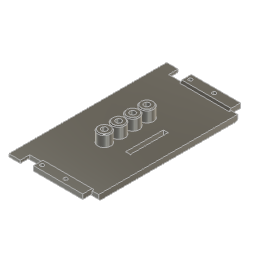
Case_Passthrough_v4 (Autodesk Fusion 360 design; units mm, degrees)
Autodesk Fusion 360 part; units mm, degrees
note: some values were not read from the file. Set by a fixed rule: which sketch regions a step uses.
sketch "Sketch1" plane through (0, 0, 0) normal (0, 0, 1) x (1, 0, 0)
  line L0 (0, 0) -> (-85, 0)
  line L1 (-85, 0) -> (-85, 147)
  line L2 (-85, 147) -> (0, 147)
  line L3 (0, 147) -> (0, 0)
  line L4 (-85, 0) -> (-85, 73.5)
  line L5 (-85, 73.5) -> (-85, 152)
  line L6 (-85, 73.5) -> (-85, -5)
  line L7 (-85, 152) -> (0, 152)
  line L8 (-85, -5) -> (0, -5)
  line L9 (-85, 152) -> (-55, 152)
  line L10 (-85, 152) -> (-30, 152)
  circle A0 centre (-55, 152) radius 2
  circle A1 centre (-30, 152) radius 2
  line L11 (-55, 152) -> (-55, -5)
  line L12 (-30, 152) -> (-30, -5)
  circle A2 centre (-55, -5) radius 2
  circle A3 centre (-30, -5) radius 2
  line L13 (-85, 147) -> (-73, 147)
  line L14 (-85, 147) -> (-59, 147)
  line L15 (-85, 147) -> (-7, 147)
  line L16 (-85, 147) -> (0, 147)
  line L17 (0, 147) -> (0, 157)
  line L18 (0, 157) -> (-85, 157)
  line L19 (-85, 157) -> (-85, 147)
  line L20 (-85, 0) -> (0, 0)
  line L21 (0, 0) -> (0, -10)
  line L22 (0, -10) -> (-85, -10)
  line L23 (-85, -10) -> (-85, 0)
  line L24 (-73, 147) -> (-73, -10)
  line L25 (-73, 147) -> (-73, 157)
  line L26 (-59, 147) -> (-59, 157)
  line L27 (-59, 147) -> (-59, -10)
  line L28 (-7, 147) -> (-7, 157)
  line L29 (-7, 147) -> (-7, -10)
  dimension "d1" = 85
  dimension "d2" = 147
  dimension "d3" = 78.5
  dimension "d4" = 78.5
  dimension "d5" = 30
  dimension "d6" = 55
  dimension "d7" = 4
  dimension "d8" = 4
  dimension "d9" = 4
  dimension "d10" = 4
  dimension "d11" = 12
  dimension "d12" = 26
  dimension "d13" = 78
  constraint horizontal L0
  constraint vertical L1
  constraint horizontal L2
  constraint vertical L3
  constraint coincident L0.start L3.end
  constraint midpoint L1 L4.end
  constraint perpendicular L2 L5
  constraint parallel L4 L6
  constraint perpendicular L5 L7
  constraint perpendicular L6 L8
  constraint perpendicular L5 L9
  constraint perpendicular L5 L10
  constraint coincident L9.end A0.centre
  constraint coincident L10.end A1.centre
  constraint coincident L8 L11.end
  constraint perpendicular L8 L11
  constraint coincident L8 L12.end
  constraint perpendicular L8 L12
  constraint coincident L11.end A2.centre
  constraint coincident L12.end A3.centre
  constraint perpendicular L1 L13
  constraint perpendicular L11 L14
  constraint perpendicular L12 L15
  constraint horizontal L16
  constraint vertical L17
  constraint horizontal L18
  constraint vertical L19
  constraint horizontal L20
  constraint vertical L21
  constraint horizontal L22
  constraint vertical L23
  constraint coincident L22 L24.end
  constraint perpendicular L22 L24
  constraint coincident L18 L25.end
  constraint perpendicular L18 L25
  constraint coincident L18 L26.end
  constraint perpendicular L18 L26
  constraint coincident L22 L27.end
  constraint perpendicular L22 L27
  constraint coincident L18 L28.end
  constraint perpendicular L18 L28
  constraint coincident L22 L29.end
  constraint perpendicular L22 L29
  measures "d1" distance of L0.start L0.end
  measures "d2" distance of L0.start L2.end
  measures "d3" distance of L4.end L5.end
  measures "d4" distance of L4.end L6.end
  measures "d5" distance of L5.end L9.end
  measures "d6" distance of L5.end L10.end
  measures "d7" diameter of A0
  measures "d8" diameter of A1
  measures "d9" diameter of A2
  measures "d10" diameter of A3
  measures "d11" distance of L1.end L13.end
  measures "d12" distance of L1.end L14.end
  measures "d13" distance of L1.end L15.end
extrude "Extrude1" add sketch "Sketch1" along normal blind 3 contours L0 L2 L3 L16 L20 L29 | L0 L8 L12 A3 L20 L29 | L0 L2 L12 L15 L16 L20 L29 | L0 L8 L11 L12 A2 A3 L20 | L0 L2 L11 L12 L15 L16 L20 | L2 L7 A1 L12 L15 L16 L28 | L8 A2 A3 L22 L27 L29 | L0 L8 L11 A2 L20 L27 | L0 L2 L11 L15 L16 L20 L27 | L2 L7 L10 A0 A1 L11 L12 L15 L16 | L7 L9 L10 A0 A1 L18 L26 L28 | L0 L2 L14 L15 L16 L20 L24 L27 | L2 L7 L9 L10 A0 L11 L15 L16 L26 | L0 L6 L8 L20 L23 L24 | L0 L1 L2 L4 L5 L6 L13 L14 L15 L16 L20 L24 | L8 L22 L23 L24 | L2 L5 L7 L9 L10 L13 L14 L15 L16 L19 L25 | L7 L9 L10 L18 L19 L25
sketch "Sketch2" plane through (0, 0, 0) normal (0, 0, 1) x (1, 0, 0)
extrude "Extrude2" add sketch "Sketch1" against normal blind 3 contours L0 L2 L3 L16 L20 L29 | L0 L2 L12 L15 L16 L20 L29 | L0 L2 L11 L12 L15 L16 L20 | L0 L2 L11 L15 L16 L20 L27 | L0 L2 L14 L15 L16 L20 L24 L27 | L0 L1 L2 L4 L5 L6 L13 L14 L15 L16 L20 L24
sketch "Sketch3" plane through (0, 0, 0) normal (0, 0, 1) x (1, 0, 0)
sketch "Sketch4" plane through (0, 0, -3) normal (0, 0, -1) x (1, 0, 0)
  line L0 (-85, 0) -> (-85, -147)
  line L1 (-85, -147) -> (0, -147)
  line L2 (0, -147) -> (0, 0)
  line L3 (0, 0) -> (-85, 0)
  line L4 (-85, 0) -> (-75, 0)
  line L5 (-75, 0) -> (-75, -10)
  line L6 (-75, -10) -> (-85, -10)
  line L7 (-85, -10) -> (-85, 0)
  line L8 (0, -147) -> (-10, -147)
  line L9 (-10, -147) -> (-10, -137)
  line L10 (-10, -137) -> (0, -137)
  line L11 (0, -137) -> (0, -147)
  line L12 (-75, -10) -> (-10, -10)
  line L13 (-10, -10) -> (-10, -137)
  line L14 (-10, -137) -> (-75, -137)
  line L15 (-75, -137) -> (-75, -10)
  dimension "d18" = 10
  dimension "d19" = 10
  dimension "d20" = 10
  dimension "d21" = 10
  constraint horizontal L4
  constraint vertical L5
  constraint horizontal L6
  constraint vertical L7
  constraint coincident L0.start L3.end
  constraint horizontal L8
  constraint vertical L9
  constraint horizontal L10
  constraint vertical L11
  constraint coincident L1.end L2.start
  constraint horizontal L12
  constraint vertical L13
  constraint horizontal L14
  constraint vertical L15
  measures "d18" distance of L0.start L4.end
  measures "d19" distance of L0.start L6.end
  measures "d20" distance of L1.end L8.end
  measures "d21" distance of L1.end L10.end
extrude "Extrude3" cut sketch "Sketch4" against normal blind 3 contours L12 L13 L14 L15
sketch "Sketch5" plane through (0, 0, 3) normal (0, 0, 1) x (-1, 0, 0)
  circle A0 centre (55, 5) radius 2
  circle A1 centre (55, -152) radius 2
  circle A2 centre (30, -152) radius 2
  circle A3 centre (30, 5) radius 2
  line L0 (73, 0) -> (59, 0)
  line L1 (59, 0) -> (59, 10)
  line L2 (59, 10) -> (7, 10)
  line L3 (7, 10) -> (7, 0)
  line L4 (7, 0) -> (0, 0)
  line L5 (0, 0) -> (0, -147)
  line L6 (0, -147) -> (7, -147)
  line L7 (7, -147) -> (7, -157)
  line L8 (7, -157) -> (59, -157)
  line L9 (59, -157) -> (59, -147)
  line L10 (59, -147) -> (73, -147)
  line L11 (73, -147) -> (73, -157)
  line L12 (73, -157) -> (85, -157)
  line L13 (85, -157) -> (85, 10)
  line L14 (85, 10) -> (73, 10)
  line L15 (73, 10) -> (73, 0)
  line L16 (0, -25) -> (45, -25)
  line L17 (45, 10) -> (45, -157)
  line L18 (45, -147) -> (45, -122)
  line L19 (45, -122) -> (44.0036, -122)
  line L20 (44.0036, -122) -> (0, -122)
  line L21 (45, 0) -> (45, -147)
  line L22 (45, -73.5) -> (0, -73.5)
  line L23 (45, -73.5) -> (45, -72.6195)
  line L24 (45, -73.5) -> (45, -66)
  line L25 (45, -66) -> (45, -51)
  line L26 (45, -66) -> (45, -81)
  line L27 (45, -81) -> (45, -96)
  circle A4 centre (45, -51) radius 3
  circle A5 centre (45, -66) radius 3
  circle A6 centre (45, -81) radius 3
  circle A7 centre (45, -96) radius 3
  dimension "d24" = 25
  dimension "d25" = 7.5
  dimension "d26" = 15
  dimension "d27" = 15
  dimension "d28" = 15
  dimension "d29" = 6
  dimension "d30" = 6
  dimension "d31" = 6
  dimension "d32" = 6
  constraint coincident L5 L16.start
  constraint perpendicular L13 L16
  constraint coincident L2 L17.start
  constraint coincident L8 L17.end
  constraint perpendicular L8 L17
  constraint coincident L17 L18.start
  constraint perpendicular L6 L18
  constraint perpendicular L17 L19
  constraint coincident L5 L20.end
  constraint perpendicular L5 L20
  constraint coincident L17 L21.start
  constraint midpoint L17 L22.start
  constraint midpoint L5 L22.end
  constraint coincident L17 L23.end
  constraint parallel L17 L23
  constraint perpendicular L22 L24
  constraint parallel L21 L25
  constraint parallel L17 L26
  constraint parallel L17 L27
  constraint coincident L25.end A4.centre
  constraint coincident L24.end L25.start
  constraint coincident L26.end L27.start
  constraint coincident L27.end A7.centre
  measures "d24" distance of L18.start L18.end
  measures "d25" distance of L22.start L24.end
  measures "d26" distance of L24.end L25.end
  measures "d27" distance of L24.end L26.end
  measures "d28" distance of L26.end L27.end
  measures "d29" diameter of A4
  measures "d30" diameter of A5
  measures "d31" diameter of A6
  measures "d32" diameter of A7
extrude "Extrude4" cut sketch "Sketch5" against normal blind 15 contours L17 L21 L25 A4 | L17 L21 L25 A4 | L17 L21 L24 L25 L26 A5 | L17 L21 L24 L25 L26 A5 | L17 L21 L26 L27 A6 | L17 L21 L26 L27 A6 | L17 L21 L27 A7 | L17 L21 L27 A7
sketch "Sketch6" plane through (0, 0, 0) normal (0, 0, 1) x (1, 0, 0)
  circle A0 centre (-45, 96) radius 7.0008
  circle A1 centre (-45, 81) radius 7.0078
  circle A2 centre (-45, 66) radius 7.0099
  circle A3 centre (-45, 51) radius 7.0057
  circle A4 centre (-45, 96) radius 3
  circle A5 centre (-45, 81) radius 3
  circle A6 centre (-45, 66) radius 3
  circle A7 centre (-45, 51) radius 3
  circle A8 centre (-45, 96) radius 3
  circle A9 centre (-45, 81) radius 3
  circle A10 centre (-45, 66) radius 3
  circle A11 centre (-45, 51) radius 3
  constraint concentric A0 A4
  constraint concentric A1 A5
  constraint concentric A2 A6
  constraint concentric A3 A7
  constraint concentric A4 A8
  constraint concentric A5 A9
  constraint concentric A2 A10
  constraint concentric A3 A11
extrude "Extrude5" add sketch "Sketch6" along normal blind 15
sketch "Sketch7" plane through (-85, 0, 0) normal (-1, 0, 0) x (0, -1, 0)
  line L0 (-157, 0) -> (-147, 0)
  line L1 (-147, 0) -> (-147, -3)
  line L2 (-147, -3) -> (0, -3)
  line L3 (0, -3) -> (0, 0)
  line L4 (0, 0) -> (10, 0)
  line L5 (10, 0) -> (10, 3)
  line L6 (10, 3) -> (-157, 3)
  line L7 (-157, 3) -> (-157, 0)
  line L8 (-51, 3) -> (-51, 15)
  line L9 (-51, 15) -> (-51, 9)
  line L10 (-51, 9) -> (-66, 9)
  line L11 (-66, 9) -> (-81, 9)
  line L12 (-81, 9) -> (-96, 9)
  circle A0 centre (-51, 9) radius 2.25
  circle A1 centre (-66, 9) radius 2.25
  circle A2 centre (-81, 9) radius 2.25
  circle A3 centre (-96, 9) radius 2.25
  dimension "d37" = 4.5
  dimension "d38" = 4.5
  dimension "d39" = 4.5
  dimension "d40" = 4.5
  constraint coincident L6 L8.start
  constraint perpendicular L6 L8
  constraint midpoint L8 L9.end
  constraint perpendicular L9 L10
  constraint perpendicular L9 L11
  constraint perpendicular L9 L12
  constraint coincident L9.end L10.start
  constraint coincident L10.end L11.start
  constraint coincident L11.end L12.start
  constraint coincident L12.end A3.centre
  measures "d37" diameter of A0
  measures "d38" diameter of A1
  measures "d39" diameter of A2
  measures "d40" diameter of A3
extrude "Extrude6" cut sketch "Sketch7" against normal blind 40 contours L8 L10 A0 | L8 L9 A0 | L8 L9 L10 A0 | L10 L11 A1 | L10 L11 A1 | L11 L12 A2 | L11 L12 A2 | A3
move_face "OffsetFaces1" offset 3 1 faces at (-20.6778, 71.149, 0)
fillet "Fillet1" radius 1 4 edges at (-51.5316, 48.4666, 15) (-51.5355, 63.4651, 15) (-51.5335, 78.4659, 15) (-51.527, 93.4684, 15)
sketch "Sketch8" plane through (0, 0, 3) normal (0, 0, 1) x (-1, 0, 0)
  circle A0 centre (45, -51) radius 7.0057
  circle A1 centre (45, -96) radius 7.0008
  circle A2 centre (45, -66) radius 7.0099
  circle A3 centre (45, -81) radius 7.0078
  circle A4 centre (55, 5) radius 2
  circle A5 centre (55, -152) radius 2
  circle A6 centre (30, -152) radius 2
  circle A7 centre (30, 5) radius 2
  line L0 (73, 0) -> (59, 0)
  line L1 (59, 0) -> (59, 10)
  line L2 (59, 10) -> (7, 10)
  line L3 (7, 10) -> (7, 0)
  line L4 (7, 0) -> (0, 0)
  line L5 (0, 0) -> (0, -147)
  line L6 (0, -147) -> (7, -147)
  line L7 (7, -147) -> (7, -157)
  line L8 (7, -157) -> (59, -157)
  line L9 (59, -157) -> (59, -147)
  line L10 (59, -147) -> (73, -147)
  line L11 (73, -147) -> (73, -157)
  line L12 (73, -157) -> (85, -157)
  line L13 (85, -157) -> (85, 10)
  line L14 (85, 10) -> (73, 10)
  line L15 (73, 10) -> (73, 0)
  line L16 (7, -147) -> (59, -147)
  line L17 (59, -147) -> (59, -157)
  line L18 (59, -157) -> (7, -157)
  line L19 (7, -157) -> (7, -147)
  line L20 (7, 10) -> (59, 10)
  line L21 (59, 10) -> (59, 0)
  line L22 (59, 0) -> (7, 0)
  line L23 (7, 0) -> (7, 10)
  circle A8 centre (30, -152) radius 2
  circle A9 centre (55, -152) radius 2
  circle A10 centre (30, 5) radius 2
  circle A11 centre (55, 5) radius 2
  constraint horizontal L16
  constraint vertical L17
  constraint horizontal L18
  constraint vertical L19
  constraint coincident L8.end L9.start
  constraint coincident L6.end L7.start
  constraint horizontal L20
  constraint vertical L21
  constraint horizontal L22
  constraint vertical L23
  constraint coincident L0.end L1.start
  constraint coincident L2.end L3.start
  constraint concentric A6 A8
  constraint concentric A5 A9
  constraint concentric A7 A10
  constraint concentric A4 A11
extrude "Extrude7" add sketch "Sketch8" along normal blind 2 contours L1 L2 L3 L20 L21 L22 L23 | L7 L8 L9 L16 L17 L18 L19
fillet "Fillet2" radius 1 4 edges at (-42.203, 52.0848, -3) (-42.203, 67.0848, -3) (-42.203, 82.0848, -3) (-42.203, 97.0848, -3)
chamfer "Chamfer1" distance 2 angle 45 2 edges at (-33, 0, 3) (-33, 147, 3)
chamfer "Chamfer2" distance 1.5 angle 45 2 edges at (-42.5, 0, -3) (-42.5, 147, -3)
sketch "Sketch9" plane through (0, 0, 3) normal (0, 0, 1) x (-1, 0, 0)
sketch "Sketch10" plane through (0, 0, -3) normal (0, 0, -1) x (1, 0, 0)
sketch "Sketch11" plane through (0, 0, 3) normal (0, 0, 1) x (-1, 0, 0)
  line L0 (85, 10) -> (85, -157)
  line L1 (85, -73.5) -> (25, -73.5)
  line L2 (25, -73.5) -> (20, -73.5)
  line L3 (20, -73.5) -> (20, -53.5)
  line L4 (20, -53.5) -> (25, -53.5)
  line L5 (25, -53.5) -> (25, -73.5)
  line L6 (25, -73.5) -> (20, -73.5)
  line L7 (20, -73.5) -> (20, -93.5)
  line L8 (20, -93.5) -> (25, -93.5)
  line L9 (25, -93.5) -> (25, -73.5)
  dimension "d52" = 167
  dimension "d53" = 5
  dimension "d54" = 20
  dimension "d55" = 20
  constraint vertical L0
  constraint midpoint L0 L1.start
  constraint perpendicular L0 L1
  constraint horizontal L2
  constraint vertical L3
  constraint horizontal L4
  constraint vertical L5
  constraint horizontal L6
  constraint vertical L7
  constraint horizontal L8
  constraint vertical L9
  measures "d52" distance of L0.start L0.end
  measures "d53" distance of L1.end L2.end
  measures "d54" distance of L1.end L4.end
  measures "d55" distance of L1.end L8.end
extrude "Extrude8" cut sketch "Sketch11" against normal blind 40
